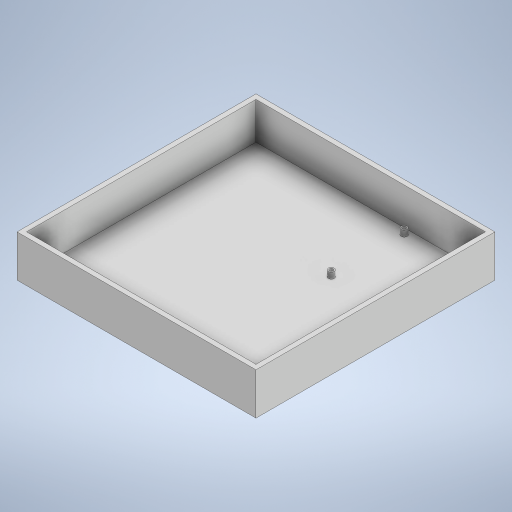
# Autodesk Inventor part: Infrared_collector
Saved by Autodesk Inventor 2024.2 (Build 282272000, 272)
## iProperties
Created: 2025-04-02
Part Number: Infrared_collector
Material: Generic
Document SubType Name: Modeling
Designer: Svend
Density: 1 g/cm^3
Appearance: Default
Author: Svend
Autodesk Inventor part; units mm, degrees
ref_plane "YZ Plane" through (0, 0, 0) normal (1, 0, 0) x (0, 1, 0)
ref_plane "XZ Plane" through (0, 0, 0) normal (0, 1, 0) x (-1, 0, 0)
ref_plane "XY Plane" through (0, 0, 0) normal (0, 0, 1) x (1, 0, 0)
sketch "Sketch1" plane through (0, 0, 0) normal (0, 1, 0) x (-1, 0, 0)
  line L0 (0, 0) -> (-200, 0)
  line L1 (-200, 0) -> (-200, 200)
  line L2 (-200, 200) -> (0, 200)
  line L3 (0, 200) -> (0, 0)
  dimension "d0" = 200
  dimension "d1" = 200
  constraints: 8 end point, 2 parallel, 1 horizontal, 1 perpendicular
  measures "d0" distance of L1.end L2.end
  measures "d1" distance of L0.end L1.end
extrude "Extrusion1" add sketch "Sketch1" along normal blind 35
sketch "Sketch2" plane through (0, 35, 0) normal (0, 1, 0) x (1, 0, 0)
  line L0 (200, 0) -> (0, 0) projected
  line L1 (0, -200) -> (200, -200) projected
  line L2 (0, 0) -> (200, 0)
  line L3 (200, 0) -> (200, -200)
  line L4 (200, -200) -> (0, -200)
  line L5 (0, -200) -> (0, 0)
  line L6 (4, -4) -> (196, -4)
  line L7 (196, -4) -> (196, -196)
  line L8 (196, -196) -> (4, -196)
  line L9 (4, -196) -> (4, -4)
  dimension "d4" = 4
  constraints: 16 end point, 4 parallel, 2 perpendicular, 1 horizontal, 3 other
  measures "d4" distance between parallel lines of L5 L9
extrude "Extrusion2" cut sketch "Sketch2" against normal blind 31 contours L6 L7 L8 L9
sketch "Sketch3" plane through (0, 4, 0) normal (0, 1, 0) x (1, 0, 0)
  line L0 (4, -4) -> (196, -4) projected
  line L1 (4, -4) -> (196, -4)
  line L2 (196, -4) -> (196, -196)
  line L3 (196, -196) -> (4, -196)
  line L4 (4, -196) -> (4, -4)
  line L5 (196, -4) -> (128, -4)
  line L6 (128, -4) -> (128, -75)
  line L7 (128, -75) -> (196, -75)
  line L8 (196, -75) -> (196, -4)
  line L9 (129, -74) -> (129, -5)
  line L10 (129, -5) -> (195, -5)
  line L11 (195, -5) -> (195, -74)
  line L12 (195, -74) -> (129, -74)
  line L13 (129, -5) -> (133, -5) construction
  line L14 (133, -5) -> (133, -9) construction
  line L15 (195, -5) -> (191, -5) construction
  line L16 (191, -5) -> (191, -9) construction
  line L17 (129, -74) -> (133, -74) construction
  line L18 (133, -74) -> (133, -70) construction
  line L19 (195, -74) -> (191, -74) construction
  line L20 (191, -74) -> (191, -70) construction
  circle A0 centre (133, -70) radius 2.5
  circle A1 centre (191, -70) radius 2.5
  circle A2 centre (191, -9) radius 2.5
  circle A3 centre (133, -9) radius 2.5
  point P0 (0, 0)
  dimension "d7" = 68
  dimension "d8" = 71
  dimension "d9" = 1
  dimension "d10" = 4
  dimension "d11" = 4
  dimension "d12" = 4
  dimension "d13" = 4
  dimension "d14" = 5
  dimension "d15" = 5
  dimension "d16" = 5
  dimension "d17" = 5
  constraints: 40 end point, 6 parallel, 6 perpendicular, 4 centre point, 4 coincident, 4 point on line, 2 horizontal, 1 vertical, 3 other
  measures "d7" distance of L7.end L6.end
  measures "d8" distance of L6.end L5.end
  measures "d9" distance between parallel lines of L6 L9
  measures "d10" distance of L9.end L13.end
  measures "d11" distance of L13.end L14.end
  measures "d12" distance of L10.end L15.end
  measures "d13" distance of L17.end L18.end
  measures "d14" diameter of A0
  measures "d15" diameter of A1
  measures "d16" diameter of A2
  measures "d17" diameter of A3
extrude "Extrusion3" add sketch "Sketch3" along normal blind 5 contours A0 | A1 | A2 | A3
sketch "Sketch4" plane through (133, 9, 70) normal (0, 1, 0) x (1, 0, 0)
  circle A0 centre (0, 0) radius 2.5
  circle A1 centre (58, 0) radius 2.5 projected
  circle A2 centre (58, 0) radius 2.5
  circle A3 centre (58, 61) radius 2.5 projected
  circle A4 centre (58, 61) radius 2.5
  circle A5 centre (0, 61) radius 2.5 projected
  circle A6 centre (0, 61) radius 2.5
  point P0 (-133, 70)
  constraints: 4 centre point, 3 coincident
hole "Hole1" at (191, 9, 9) at (133, 9, 9) at (133, 9, 70) at (191, 9, 70) direction (0, -1, 0) diameter 3 depth 8 tip angle 118
body "Solid1"
